# Autodesk Inventor part: Zahnriemen
Saved by Autodesk Inventor 2016 (Build 200138000, 138)
## iProperties
Created: 2015-08-25
Part Number: Zahnriemen
Material: Rubber
Document SubType Name: Modeling
Designer: 4ndreas
Density: 0.93 g/cm^3
Appearance: Rubber - Black - Version 1.1
Mass: 0.82026 g
Surface Area: 32.34 cm^2
Volume: 0.882 cm^3
CustomPartVersion: 1
Author: 4ndreas
Autodesk Inventor part; units mm, degrees
sketch "Skizzenpfad" plane through (0, 0, 0) normal (0, 0, 1) x (1, 0, 0)
  arc A0 (-17.0407, -68.5514) -> (-10.624, -74.7337) centre (-10.6771, -68.3677) ccw
  arc A1 (19.0965, 2.7477) -> (-19.0906, 2.4822) centre (0, 3.0331) ccw
  arc A2 (11.7228, -74.547) -> (18.0351, -68.2761) centre (11.6696, -68.181) ccw
  line L0 (11.7228, -74.547) -> (-10.624, -74.7337)
  line L1 (-17.0407, -68.5514) -> (-19.0906, 2.4822)
  line L2 (19.0965, 2.7477) -> (18.0351, -68.2761)
  constraints: 6 end point, 6 point on circle, 3 centre point
ref_plane "Querschnittsebene" through (-10.624, -74.7337, 0) normal (1, 0.0084, 0) x (0, 0, 1)
ref_plane "Arbeitsebene2" through (-10.6771, -68.3677, 0) normal (-1, 0, 0) x (0, 0, 1)
ref_plane "Arbeitsebene3" through (0, 3.0331, 0) normal (-0.056, -0.9984, 0) x (0, 0, 1)
ref_plane "Arbeitsebene4" through (11.6696, -68.181, 0) normal (0.3604, 0.9328, 0) x (0, 0, 1)
sketch "Querschnitt" plane through (-10.624, -74.7337, 0) normal (1, 0.0084, 0) x (0, 0, 1)
  line L0 (-3, 0.3) -> (3, 0.3)
  line L1 (3, 0.3) -> (3, -0.3)
  line L2 (3, -0.3) -> (-3, -0.3)
  line L3 (-3, -0.3) -> (-3, 0.3)
  line L4 (-3, 0) -> (3, 0) construction
  point P0 (0, 0)
  point P1 (0, 0)
  dimension "d0" = 6
  dimension "d4" = 0.3
  dimension "d5" = 0.3
  constraints: 10 end point, 3 midpoint, 2 parallel, 1 coincident, 1 horizontal, 1 perpendicular, 1 other
  measures "d0" distance between parallel lines of L1 L3
  measures "d4" distance between parallel lines of L2 L4
  measures "d5" distance between parallel lines of L4 L0
sweep "Riemen" add profiles "Querschnitt" path "Skizzenpfad"
equation "\"d0\" = da_B"
equation "\"d4\" = da_a"
equation "\"d5\" = da_a2"
equation "\"da_B\" = 6"
equation "\"da_pb\" = 2.5"
equation "\"da_L\" = 245"
equation "\"da_a\" = 0.3"
equation "\"da_S\" = 1.5"
equation "\"da_Beta\" = 20deg"
equation "\"da_Ht\" = 0.7"
equation "\"da_H\" = 1.3"
equation "\"da_a2\" = 0.3"
body "Solid1"
